naoise_thing (Autodesk Fusion 360 design; units mm, degrees)
Autodesk Fusion 360 part; units mm, degrees
note: some values were not read from the file. Set by a fixed rule: which sketch regions a step uses.
(part 1 of 2)
sketch "Sketch2" plane through (0, 0, 0) normal (0, 0, 1) x (1, 0, 0)
  spline S0 degree 3 poles (35.719, -1.0848) (35.583, -1.8378) (35.7119, -15.8578) (35.8563, -16.002) knots 0 0 0 0 1 1 1 1
  spline S1 degree 3 poles (35.8563, -16.002) (36.0722, -16.2179) (69.5076, -16.2584) (69.8021, -16.0433) knots 0 0 0 0 1 1 1 1
  spline S2 degree 3 poles (69.8021, -16.0433) (70.0037, -15.8956) (70.0088, -15.7107) (70.0088, -8.4275) knots 0 0 0 0 1 1 1 1
  spline S3 degree 3 poles (70.0088, -8.4275) (70.0088, 0.3215) (70.0741, -0.0561) (68.8446, -1.7161) knots 0 0 0 0 1 1 1 1
  spline S4 degree 3 poles (68.8446, -1.7161) (64.4631, -7.6311) (59.6874, -7.6798) (54.1131, -1.8661) knots 0 0 0 0 1 1 1 1
  spline S5 degree 3 poles (54.1131, -1.8661) (53.5197, -1.2472) (52.9609, -0.7408) (52.8712, -0.7408) knots 0 0 0 0 1 1 1 1
  spline S6 degree 3 poles (52.8712, -0.7408) (52.7815, -0.7408) (52.1002, -1.3499) (51.3572, -2.0944) knots 0 0 0 0 1 1 1 1
  spline S7 degree 3 poles (51.3572, -2.0944) (45.7435, -7.7192) (41.5531, -7.6258) (36.9001, -1.7727) knots 0 0 0 0 1 1 1 1
  spline S8 degree 3 poles (36.9001, -1.7727) (36.0177, -0.6628) (35.8166, -0.5456) (35.719, -1.0848) knots 0 0 0 0 1 1 1 1
  spline S9 degree 3 poles (0.635, -11.6292) (0.223, -11.7446) (0.2588, -12.0764) (0.7948, -13.1146) knots 0 0 0 0 1 1 1 1
  spline S10 degree 3 poles (0.7948, -13.1146) (2.1296, -15.6988) (3.7576, -16.9738) (6.2135, -17.3577) knots 0 0 0 0 1 1 1 1
  spline S11 degree 3 poles (6.2135, -17.3577) (7.3075, -17.5289) (7.2747, -17.504) (7.5221, -18.342) knots 0 0 0 0 1 1 1 1
  spline S12 degree 3 poles (7.5221, -18.342) (8.2973, -20.968) (9.7838, -22.1623) (12.7302, -22.5269) knots 0 0 0 0 1 1 1 1
  spline S13 degree 3 poles (12.7302, -22.5269) (13.7266, -22.6502) (13.756, -22.6727) (14.3089, -23.7358) knots 0 0 0 0 1 1 1 1
  spline S14 degree 3 poles (14.3089, -23.7358) (15.7255, -26.4583) (17.1659, -26.9026) (24.6592, -26.9285) knots 0 0 0 0 1 1 1 1
  line L0 (24.6592, -26.9285) -> (29.3687, -26.9449)
  line L1 (29.3688, -26.9449) -> (30.4469, -27.6577)
  spline S15 degree 3 poles (30.4469, -27.6577) (33.8122, -29.8826) (38.332, -30.8367) (42.83, -30.2715) knots 0 0 0 0 1 1 1 1
  spline S16 degree 3 poles (42.83, -30.2715) (44.7186, -30.0342) (44.7204, -29.8995) (42.8464, -29.0565) knots 0 0 0 0 1 1 1 1
  spline S17 degree 3 poles (42.8464, -29.0565) (36.3696, -26.1432) (32.2559, -21.2281) (29.5241, -13.1397) knots 0 0 0 0 1 1 1 1
  spline S18 degree 3 poles (29.5241, -13.1397) (29.2978, -12.4703) (29.0378, -11.8475) (28.9459, -11.7557) knots 0 0 0 0 1 1 1 1
  spline S19 degree 3 poles (28.9459, -11.7557) (28.7689, -11.5784) (1.2562, -11.4557) (0.635, -11.6292) knots 0 0 0 0 1 1 1 1
  spline S20 degree 3 poles (77.0705, -11.611) (76.7252, -11.6771) (76.594, -11.9293) (75.9828, -13.6993) knots 0 0 0 0 1 1 1 1
  spline S21 degree 3 poles (75.9828, -13.6993) (73.2996, -21.4731) (69.0594, -26.361) (62.5277, -29.2105) knots 0 0 0 0 1 1 1 1
  spline S22 degree 3 poles (62.5277, -29.2105) (61.0055, -29.8744) (61.0529, -30.0667) (62.7854, -30.2601) knots 0 0 0 0 1 1 1 1
  spline S23 degree 3 poles (62.7854, -30.2601) (67.6685, -30.8044) (71.9122, -29.9088) (75.3533, -27.6072) knots 0 0 0 0 1 1 1 1
  line L2 (75.3533, -27.6072) -> (76.3588, -26.9346)
  line L3 (76.3588, -26.9346) -> (79.7454, -26.9661)
  spline S24 degree 3 poles (79.7454, -26.9661) (88.0734, -27.0433) (90.0023, -26.4845) (91.503, -23.5596) knots 0 0 0 0 1 1 1 1
  spline S25 degree 3 poles (91.503, -23.5596) (91.9636, -22.6618) (92.044, -22.6121) (93.222, -22.4922) knots 0 0 0 0 1 1 1 1
  spline S26 degree 3 poles (93.222, -22.4922) (95.7363, -22.2366) (97.354, -20.9555) (98.0726, -18.651) knots 0 0 0 0 1 1 1 1
  spline S27 degree 3 poles (98.0726, -18.651) (98.4165, -17.5477) (98.4499, -17.5159) (99.4143, -17.3725) knots 0 0 0 0 1 1 1 1
  spline S28 degree 3 poles (99.4143, -17.3725) (101.9715, -16.9923) (103.7812, -15.5445) (105.0568, -12.8585) knots 0 0 0 0 1 1 1 1
  spline S29 degree 3 poles (105.0568, -12.8585) (105.4714, -11.9854) (105.4783, -11.738) (105.092, -11.6303) knots 0 0 0 0 1 1 1 1
  spline S30 degree 3 poles (105.092, -11.6303) (104.8102, -11.552) (77.4766, -11.5329) (77.0705, -11.611) knots 0 0 0 0 1 1 1 1
  spline S31 degree 3 poles (52.3581, -27.8543) (51.9438, -28.589) (48.2476, -35.5724) (47.3265, -37.3605) knots 0 0 0 0 1 1 1 1
  spline S32 degree 3 poles (47.3265, -37.3605) (46.3479, -39.2607) (46.3468, -39.1938) (47.3644, -39.8854) knots 0 0 0 0 1 1 1 1
  spline S33 degree 3 poles (47.3644, -39.8854) (49.407, -41.2737) (49.8475, -42.7553) (49.8475, -48.2391) knots 0 0 0 0 1 1 1 1
  spline S34 degree 3 poles (49.8475, -48.2391) (49.8475, -52.5754) (49.9795, -52.1877) (48.4182, -52.4357) knots 0 0 0 0 1 1 1 1
  spline S35 degree 3 poles (48.4182, -52.4357) (36.6948, -54.2975) (27.8365, -64.1128) (27.141, -76.0116) knots 0 0 0 0 1 1 1 1
  spline S36 degree 3 poles (27.141, -76.0116) (27.0357, -77.8134) (27.6042, -77.6293) (22.1541, -77.6256) knots 0 0 0 0 1 1 1 1
  spline S37 degree 3 poles (22.1541, -77.6256) (15.6213, -77.6208) (14.2327, -77.2231) (12.8855, -74.9705) knots 0 0 0 0 1 1 1 1
  spline S38 degree 3 poles (12.8855, -74.9705) (12.391, -74.1437) (12.4203, -74.1394) (10.0756, -75.3867) knots 0 0 0 0 1 1 1 1
  spline S39 degree 3 poles (10.0756, -75.3867) (8.9286, -75.9965) (7.3237, -76.8287) (6.5088, -77.2356) knots 0 0 0 0 1 1 1 1
  spline S40 degree 3 poles (6.5088, -77.2356) (4.3691, -78.3042) (0.8178, -80.2058) (0.6506, -80.3727) knots 0 0 0 0 1 1 1 1
  spline S41 degree 3 poles (0.6506, -80.3727) (0.3257, -80.6966) (0.6289, -80.921) (3.3086, -82.3394) knots 0 0 0 0 1 1 1 1
  spline S42 degree 3 poles (3.3086, -82.3394) (4.7776, -83.117) (6.9321, -84.2619) (8.0963, -84.8836) knots 0 0 0 0 1 1 1 1
  spline S43 degree 3 poles (8.0963, -84.8836) (12.5838, -87.2808) (12.3521, -87.2112) (12.8865, -86.3177) knots 0 0 0 0 1 1 1 1
  spline S44 degree 3 poles (12.8865, -86.3177) (13.5485, -85.2106) (14.832, -84.3254) (16.4571, -83.8544) knots 0 0 0 0 1 1 1 1
  spline S45 degree 3 poles (16.4571, -83.8544) (17.5273, -83.544) (27.5381, -83.5073) (27.7995, -83.8126) knots 0 0 0 0 1 1 1 1
  spline S46 degree 3 poles (27.7995, -83.8126) (28.6538, -84.8103) (28.806, -87.4985) (28.1056, -89.2201) knots 0 0 0 0 1 1 1 1
  spline S47 degree 3 poles (28.1056, -89.2201) (27.4325, -90.8748) (27.0375, -93.0585) (27.201, -94.2189) knots 0 0 0 0 1 1 1 1
  spline S48 degree 3 poles (27.201, -94.2189) (27.5804, -96.91) (34.4808, -102.4467) (37.4555, -102.4467) knots 0 0 0 0 1 1 1 1
  spline S49 degree 3 poles (37.4555, -102.4467) (39.3348, -102.4467) (40.9678, -99.7635) (41.8999, -95.1442) knots 0 0 0 0 1 1 1 1
  spline S50 degree 3 poles (41.8999, -95.1442) (42.8593, -90.3891) (42.3669, -88.6473) (39.5851, -86.9574) knots 0 0 0 0 1 1 1 1
  spline S51 degree 3 poles (39.5851, -86.9574) (37.9746, -85.979) (36.8218, -84.2939) (37.3803, -83.7353) knots 0 0 0 0 1 1 1 1
  spline S52 degree 3 poles (37.3803, -83.7353) (37.6208, -83.4948) (49.4525, -83.5589) (49.6723, -83.8017) knots 0 0 0 0 1 1 1 1
  spline S53 degree 3 poles (49.6723, -83.8017) (49.9007, -84.0542) (49.9388, -98.6692) (49.7118, -98.9613) knots 0 0 0 0 1 1 1 1
  spline S54 degree 3 poles (49.7118, -98.9613) (49.6409, -99.0523) (49.1305, -99.4521) (48.5775, -99.8495) knots 0 0 0 0 1 1 1 1
  spline S55 degree 3 poles (48.5775, -99.8495) (42.4288, -104.2681) (38.5662, -110.0365) (37.342, -116.6283) knots 0 0 0 0 1 1 1 1
  spline S56 degree 3 poles (37.342, -116.6283) (37.1642, -117.5861) (37.1652, -121.3281) (37.3436, -122.4492) knots 0 0 0 0 1 1 1 1
  spline S57 degree 3 poles (37.3436, -122.4492) (38.309, -128.5137) (42.2148, -134.9542) (48.2854, -140.4911) knots 0 0 0 0 1 1 1 1
  spline S58 degree 3 poles (48.2854, -140.4911) (49.027, -141.1676) (49.6819, -141.8109) (49.7406, -141.9206) knots 0 0 0 0 1 1 1 1
  spline S59 degree 3 poles (49.7406, -141.9206) (49.938, -142.2892) (49.8811, -158.2782) (49.6792, -159.2564) knots 0 0 0 0 1 1 1 1
  spline S60 degree 3 poles (49.6792, -159.2564) (49.2913, -161.1344) (48.4841, -162.4113) (47.1736, -163.2212) knots 0 0 0 0 1 1 1 1
  spline S61 degree 3 poles (47.1736, -163.2212) (46.291, -163.7665) (46.2367, -163.5546) (48.2158, -167.3032) knots 0 0 0 0 1 1 1 1
  spline S62 degree 3 poles (48.2158, -167.3032) (49.1892, -169.1473) (50.4865, -171.6087) (51.0987, -172.7729) knots 0 0 0 0 1 1 1 1
  spline S63 degree 3 poles (51.0987, -172.7729) (52.682, -175.7839) (52.7915, -175.9355) (53.1043, -175.551) knots 0 0 0 0 1 1 1 1
  spline S64 degree 3 poles (53.1043, -175.551) (53.2855, -175.328) (59.1383, -164.2084) (59.163, -164.0403) knots 0 0 0 0 1 1 1 1
  spline S65 degree 3 poles (59.163, -164.0403) (59.2132, -163.6961) (59.1338, -163.5995) (58.4277, -163.1471) knots 0 0 0 0 1 1 1 1
  spline S66 degree 3 poles (58.4277, -163.1471) (57.6789, -162.6672) (57.0645, -161.9695) (56.6327, -161.109) knots 0 0 0 0 1 1 1 1
  spline S67 degree 3 poles (56.6327, -161.109) (56.2655, -160.3775) (56.3258, -160.1044) (57.0807, -159.0797) knots 0 0 0 0 1 1 1 1
  spline S68 degree 3 poles (57.0807, -159.0797) (58.5393, -157.0993) (59.1905, -155.9229) (59.794, -154.1772) knots 0 0 0 0 1 1 1 1
  spline S69 degree 3 poles (59.794, -154.1772) (61.8601, -148.2013) (60.8065, -143.0586) (56.1922, -136.5957) knots 0 0 0 0 1 1 1 1
  line L4 (56.1922, -136.5957) -> (55.8271, -136.0845)
  line L5 (55.8271, -136.0845) -> (55.8271, -121.144)
  spline S70 degree 3 poles (55.8271, -121.144) (55.8271, -109.8153) (55.8575, -106.1508) (55.9525, -105.9852) knots 0 0 0 0 1 1 1 1
  spline S71 degree 3 poles (55.9525, -105.9852) (56.0774, -105.768) (58.6944, -103.9831) (62.23, -101.7042) knots 0 0 0 0 1 1 1 1
  spline S72 degree 3 poles (62.23, -101.7042) (70.1106, -96.6245) (74.0892, -91.9438) (76.2611, -85.1958) knots 0 0 0 0 1 1 1 1
  spline S73 degree 3 poles (76.2611, -85.1958) (76.835, -83.4139) (76.0812, -83.5922) (82.859, -83.634) knots 0 0 0 0 1 1 1 1
  spline S74 degree 3 poles (82.859, -83.634) (88.5187, -83.6689) (88.6516, -83.6745) (89.4284, -83.911) knots 0 0 0 0 1 1 1 1
  spline S75 degree 3 poles (89.4284, -83.911) (91.0037, -84.3907) (92.093, -85.1551) (92.774, -86.2584) knots 0 0 0 0 1 1 1 1
  spline S76 degree 3 poles (92.774, -86.2584) (93.3916, -87.2591) (92.3584, -87.6665) (101.5214, -82.8074) knots 0 0 0 0 1 1 1 1
  spline S77 degree 3 poles (101.5214, -82.8074) (105.0269, -80.9485) (105.3714, -80.7164) (105.1039, -80.3942) knots 0 0 0 0 1 1 1 1
  spline S78 degree 3 poles (105.1039, -80.3942) (105.0425, -80.3201) (103.6455, -79.5552) (101.9995, -78.694) knots 0 0 0 0 1 1 1 1
  spline S79 degree 3 poles (101.9995, -78.694) (92.4428, -73.6949) (93.3447, -74.0624) (92.8367, -74.9612) knots 0 0 0 0 1 1 1 1
  spline S80 degree 3 poles (92.8367, -74.9612) (91.5382, -77.2589) (89.7731, -77.7116) (82.3156, -77.6594) knots 0 0 0 0 1 1 1 1
  spline S81 degree 3 poles (82.3156, -77.6594) (77.0308, -77.6227) (77.5811, -77.8288) (77.4594, -75.8407) knots 0 0 0 0 1 1 1 1
  spline S82 degree 3 poles (77.4594, -75.8407) (76.7593, -64.4001) (68.4755, -54.9127) (57.1704, -52.6031) knots 0 0 0 0 1 1 1 1
  spline S83 degree 3 poles (57.1704, -52.6031) (55.7048, -52.3039) (55.8266, -52.6957) (55.8308, -48.2822) knots 0 0 0 0 1 1 1 1
  spline S84 degree 3 poles (55.8308, -48.2822) (55.8358, -42.7199) (56.4335, -40.885) (58.6317, -39.6811) knots 0 0 0 0 1 1 1 1
  spline S85 degree 3 poles (58.6317, -39.6811) (59.4778, -39.2176) (59.8609, -40.1143) (54.4724, -29.9508) knots 0 0 0 0 1 1 1 1
  spline S86 degree 3 poles (54.4724, -29.9508) (52.9656, -27.1084) (52.8458, -26.9896) (52.3581, -27.8543) knots 0 0 0 0 1 1 1 1
  spline S87 degree 3 poles (49.6811, -63.1373) (49.9203, -63.3762) (49.9356, -77.0972) (49.6972, -77.4234) knots 0 0 0 0 1 1 1 1
  spline S88 degree 3 poles (49.6972, -77.4234) (49.5041, -77.6877) (37.2189, -77.8021) (36.7242, -77.5441) knots 0 0 0 0 1 1 1 1
  spline S89 degree 3 poles (36.7242, -77.5441) (35.9989, -77.166) (36.9401, -73.3586) (38.3775, -70.8554) knots 0 0 0 0 1 1 1 1
  spline S90 degree 3 poles (57.8908, -63.6773) (63.0642, -65.5854) (67.0576, -70.3741) (68.0736, -75.8881) knots 0 0 0 0 1 1 1 1
  spline S91 degree 3 poles (68.0736, -75.8881) (68.321, -77.2313) (68.2993, -77.421) (67.881, -77.5801) knots 0 0 0 0 1 1 1 1
  spline S92 degree 3 poles (67.881, -77.5801) (67.3201, -77.7933) (56.2385, -77.6624) (56.016, -77.4398) knots 0 0 0 0 1 1 1 1
  spline S93 degree 3 poles (56.016, -77.4398) (55.7551, -77.179) (55.7197, -63.6619) (55.979, -63.3495) knots 0 0 0 0 1 1 1 1
  spline S94 degree 3 poles (55.979, -63.3495) (56.1729, -63.1158) (56.5393, -63.1788) (57.8908, -63.6773) knots 0 0 0 0 1 1 1 1
  spline S95 degree 3 poles (67.3095, -83.7663) (67.6767, -84.2089) (65.918, -87.6308) (64.3448, -89.535) knots 0 0 0 0 1 1 1 1
  spline S96 degree 3 poles (57.4818, -94.9415) (56.1676, -95.6654) (56.0155, -95.6757) (55.8543, -95.0534) knots 0 0 0 0 1 1 1 1
  spline S97 degree 3 poles (55.8543, -95.0534) (55.6953, -94.4396) (55.8046, -83.9851) (55.9723, -83.7832) knots 0 0 0 0 1 1 1 1
  spline S98 degree 3 poles (55.9723, -83.7832) (56.1827, -83.5298) (67.0997, -83.5136) (67.3095, -83.7663) knots 0 0 0 0 1 1 1 1
  spline S99 degree 3 poles (47.0956, -117.9573) (47.6329, -115.5229) (49.1337, -112.3511) (49.6647, -112.5281) knots 0 0 0 0 1 1 1 1
  spline S100 degree 3 poles (49.6647, -112.5281) (49.7655, -112.5617) (49.8007, -114.3624) (49.8218, -120.5659) knots 0 0 0 0 1 1 1 1
  line L6 (0, -88.0004) -> (0, -176.0008)
  line L7 (0, -176.0008) -> (52.9167, -176.0008)
  line L8 (52.9167, -176.0008) -> (105.8333, -176.0008)
  line L9 (105.8333, -176.0008) -> (105.8333, -88.0004)
  line L10 (105.8333, -88.0004) -> (105.8333, 0)
  line L11 (105.8333, 0) -> (52.9167, 0)
  line L12 (52.9167, 0) -> (0, 0)
  line L13 (0, 0) -> (0, -88.0004)
  spline S101 degree 3 poles (36.9001, -1.7727) (41.5531, -7.6258) (45.7435, -7.7192) (51.3572, -2.0944) knots 0 0 0 0 1 1 1 1
  spline S102 degree 3 poles (51.3572, -2.0944) (52.1002, -1.3499) (52.7815, -0.7408) (52.8712, -0.7408) knots 0 0 0 0 1 1 1 1
  spline S103 degree 3 poles (52.8712, -0.7408) (52.9609, -0.7408) (53.5197, -1.2472) (54.1131, -1.8661) knots 0 0 0 0 1 1 1 1
  spline S104 degree 3 poles (54.1131, -1.8661) (59.6874, -7.6798) (64.4631, -7.6311) (68.8446, -1.7161) knots 0 0 0 0 1 1 1 1
  spline S105 degree 3 poles (68.8446, -1.7161) (70.0741, -0.0561) (70.0088, 0.3215) (70.0088, -8.4275) knots 0 0 0 0 1 1 1 1
  spline S106 degree 3 poles (70.0088, -8.4275) (70.0088, -15.7107) (70.0037, -15.8956) (69.8021, -16.0433) knots 0 0 0 0 1 1 1 1
  spline S107 degree 3 poles (69.8021, -16.0433) (69.5076, -16.2584) (36.0722, -16.2179) (35.8563, -16.002) knots 0 0 0 0 1 1 1 1
  spline S108 degree 3 poles (35.8563, -16.002) (35.7119, -15.8578) (35.583, -1.8378) (35.719, -1.0848) knots 0 0 0 0 1 1 1 1
  spline S109 degree 3 poles (35.719, -1.0848) (35.8166, -0.5456) (36.0177, -0.6628) (36.9001, -1.7727) knots 0 0 0 0 1 1 1 1
  spline S110 degree 3 poles (28.9459, -11.7557) (29.0378, -11.8475) (29.2978, -12.4703) (29.5241, -13.1397) knots 0 0 0 0 1 1 1 1
  spline S111 degree 3 poles (29.5241, -13.1397) (32.2559, -21.2281) (36.3696, -26.1432) (42.8464, -29.0565) knots 0 0 0 0 1 1 1 1
  spline S112 degree 3 poles (42.8464, -29.0565) (44.7204, -29.8995) (44.7186, -30.0342) (42.83, -30.2715) knots 0 0 0 0 1 1 1 1
  spline S113 degree 3 poles (42.83, -30.2715) (38.332, -30.8367) (33.8122, -29.8826) (30.4469, -27.6577) knots 0 0 0 0 1 1 1 1
  line L14 (30.4469, -27.6577) -> (29.3688, -26.9449)
  line L15 (29.3688, -26.9449) -> (24.6592, -26.9285)
  spline S114 degree 3 poles (24.6592, -26.9285) (17.1659, -26.9026) (15.7255, -26.4583) (14.3089, -23.7358) knots 0 0 0 0 1 1 1 1
  spline S115 degree 3 poles (14.3089, -23.7358) (13.756, -22.6727) (13.7266, -22.6502) (12.7302, -22.5269) knots 0 0 0 0 1 1 1 1
  spline S116 degree 3 poles (12.7302, -22.5269) (9.7838, -22.1623) (8.2973, -20.968) (7.5221, -18.342) knots 0 0 0 0 1 1 1 1
  spline S117 degree 3 poles (7.5221, -18.342) (7.2747, -17.504) (7.3075, -17.5289) (6.2135, -17.3577) knots 0 0 0 0 1 1 1 1
  spline S118 degree 3 poles (6.2135, -17.3577) (3.7576, -16.9738) (2.1296, -15.6988) (0.7948, -13.1146) knots 0 0 0 0 1 1 1 1
  spline S119 degree 3 poles (0.7948, -13.1146) (0.2588, -12.0764) (0.223, -11.7446) (0.635, -11.6292) knots 0 0 0 0 1 1 1 1
  spline S120 degree 3 poles (0.635, -11.6292) (1.2562, -11.4557) (28.7689, -11.5784) (28.9459, -11.7557) knots 0 0 0 0 1 1 1 1
  spline S121 degree 3 poles (105.092, -11.6303) (105.4783, -11.738) (105.4714, -11.9854) (105.0568, -12.8585) knots 0 0 0 0 1 1 1 1
  spline S122 degree 3 poles (105.0568, -12.8585) (103.7812, -15.5445) (101.9715, -16.9923) (99.4143, -17.3725) knots 0 0 0 0 1 1 1 1
  spline S123 degree 3 poles (99.4143, -17.3725) (98.4499, -17.5159) (98.4165, -17.5477) (98.0726, -18.651) knots 0 0 0 0 1 1 1 1
  spline S124 degree 3 poles (98.0726, -18.651) (97.354, -20.9555) (95.7363, -22.2366) (93.222, -22.4922) knots 0 0 0 0 1 1 1 1
  spline S125 degree 3 poles (93.222, -22.4922) (92.044, -22.6121) (91.9636, -22.6618) (91.503, -23.5596) knots 0 0 0 0 1 1 1 1
  spline S126 degree 3 poles (91.503, -23.5596) (90.0023, -26.4845) (88.0734, -27.0433) (79.7454, -26.9661) knots 0 0 0 0 1 1 1 1
  line L16 (79.7454, -26.9661) -> (76.3588, -26.9346)
  line L17 (76.3588, -26.9346) -> (75.3533, -27.6072)
  spline S127 degree 3 poles (75.3533, -27.6072) (71.9122, -29.9088) (67.6685, -30.8044) (62.7854, -30.2601) knots 0 0 0 0 1 1 1 1
  spline S128 degree 3 poles (62.7854, -30.2601) (61.0529, -30.0667) (61.0055, -29.8744) (62.5277, -29.2105) knots 0 0 0 0 1 1 1 1
  spline S129 degree 3 poles (62.5277, -29.2105) (69.0594, -26.361) (73.2996, -21.4731) (75.9828, -13.6993) knots 0 0 0 0 1 1 1 1
  spline S130 degree 3 poles (75.9828, -13.6993) (76.594, -11.9293) (76.7252, -11.6771) (77.0705, -11.611) knots 0 0 0 0 1 1 1 1
  spline S131 degree 3 poles (77.0705, -11.611) (77.4766, -11.5329) (104.8102, -11.552) (105.092, -11.6303) knots 0 0 0 0 1 1 1 1
  spline S132 degree 3 poles (54.4724, -29.9508) (59.8609, -40.1143) (59.4778, -39.2176) (58.6317, -39.6811) knots 0 0 0 0 1 1 1 1
  spline S133 degree 3 poles (58.6317, -39.6811) (56.4335, -40.885) (55.8358, -42.7199) (55.8308, -48.2822) knots 0 0 0 0 1 1 1 1
  spline S134 degree 3 poles (55.8308, -48.2822) (55.8266, -52.6957) (55.7048, -52.3039) (57.1704, -52.6031) knots 0 0 0 0 1 1 1 1
  spline S135 degree 3 poles (57.1704, -52.6031) (68.4755, -54.9127) (76.7593, -64.4001) (77.4594, -75.8407) knots 0 0 0 0 1 1 1 1
  spline S136 degree 3 poles (77.4594, -75.8407) (77.5811, -77.8288) (77.0308, -77.6227) (82.3156, -77.6594) knots 0 0 0 0 1 1 1 1
  spline S137 degree 3 poles (82.3156, -77.6594) (89.7731, -77.7116) (91.5382, -77.2589) (92.8367, -74.9612) knots 0 0 0 0 1 1 1 1
  spline S138 degree 3 poles (92.8367, -74.9612) (93.3447, -74.0624) (92.4428, -73.6949) (101.9995, -78.694) knots 0 0 0 0 1 1 1 1
  spline S139 degree 3 poles (101.9995, -78.694) (103.6455, -79.5552) (105.0425, -80.3201) (105.1039, -80.3942) knots 0 0 0 0 1 1 1 1
  spline S140 degree 3 poles (105.1039, -80.3942) (105.3714, -80.7164) (105.0269, -80.9485) (101.5214, -82.8074) knots 0 0 0 0 1 1 1 1
  spline S141 degree 3 poles (101.5214, -82.8074) (92.3584, -87.6665) (93.3916, -87.2591) (92.774, -86.2584) knots 0 0 0 0 1 1 1 1
  spline S142 degree 3 poles (92.774, -86.2584) (92.093, -85.1551) (91.0037, -84.3907) (89.4284, -83.911) knots 0 0 0 0 1 1 1 1
  spline S143 degree 3 poles (89.4284, -83.911) (88.6516, -83.6745) (88.5187, -83.6689) (82.859, -83.634) knots 0 0 0 0 1 1 1 1
  spline S144 degree 3 poles (82.859, -83.634) (76.0812, -83.5922) (76.835, -83.4139) (76.2611, -85.1958) knots 0 0 0 0 1 1 1 1
  spline S145 degree 3 poles (76.2611, -85.1958) (74.0892, -91.9438) (70.1106, -96.6245) (62.23, -101.7042) knots 0 0 0 0 1 1 1 1
  spline S146 degree 3 poles (62.23, -101.7042) (58.6944, -103.9831) (56.0774, -105.768) (55.9525, -105.9852) knots 0 0 0 0 1 1 1 1
  spline S147 degree 3 poles (55.9525, -105.9852) (55.8575, -106.1508) (55.8271, -109.8153) (55.8271, -121.144) knots 0 0 0 0 1 1 1 1
  line L18 (55.8271, -121.144) -> (55.8271, -136.0845)
  line L19 (55.8271, -136.0845) -> (56.1922, -136.5957)
  spline S148 degree 3 poles (56.1922, -136.5957) (60.8065, -143.0586) (61.8601, -148.2013) (59.794, -154.1772) knots 0 0 0 0 1 1 1 1
  spline S149 degree 3 poles (59.794, -154.1772) (59.1905, -155.9229) (58.5393, -157.0993) (57.0807, -159.0797) knots 0 0 0 0 1 1 1 1
  spline S150 degree 3 poles (57.0807, -159.0797) (56.3258, -160.1044) (56.2655, -160.3775) (56.6327, -161.109) knots 0 0 0 0 1 1 1 1
  spline S151 degree 3 poles (56.6327, -161.109) (57.0645, -161.9695) (57.6789, -162.6672) (58.4277, -163.1471) knots 0 0 0 0 1 1 1 1
  spline S152 degree 3 poles (58.4277, -163.1471) (59.1338, -163.5995) (59.2132, -163.6961) (59.163, -164.0403) knots 0 0 0 0 1 1 1 1
  spline S153 degree 3 poles (59.163, -164.0403) (59.1383, -164.2084) (53.2855, -175.328) (53.1043, -175.551) knots 0 0 0 0 1 1 1 1
  spline S154 degree 3 poles (53.1043, -175.551) (52.7915, -175.9355) (52.682, -175.7839) (51.0987, -172.7729) knots 0 0 0 0 1 1 1 1
  spline S155 degree 3 poles (51.0987, -172.7729) (50.4865, -171.6087) (49.1892, -169.1473) (48.2158, -167.3032) knots 0 0 0 0 1 1 1 1
  spline S156 degree 3 poles (48.2158, -167.3032) (46.2367, -163.5546) (46.291, -163.7665) (47.1736, -163.2212) knots 0 0 0 0 1 1 1 1
  spline S157 degree 3 poles (47.1736, -163.2212) (48.4841, -162.4113) (49.2913, -161.1344) (49.6792, -159.2564) knots 0 0 0 0 1 1 1 1
  spline S158 degree 3 poles (49.6792, -159.2564) (49.8811, -158.2782) (49.938, -142.2892) (49.7406, -141.9206) knots 0 0 0 0 1 1 1 1
  spline S159 degree 3 poles (49.7406, -141.9206) (49.6819, -141.8109) (49.027, -141.1676) (48.2854, -140.4911) knots 0 0 0 0 1 1 1 1
  spline S160 degree 3 poles (48.2854, -140.4911) (42.2148, -134.9542) (38.309, -128.5137) (37.3436, -122.4492) knots 0 0 0 0 1 1 1 1
  spline S161 degree 3 poles (37.3436, -122.4492) (37.1652, -121.3281) (37.1642, -117.5861) (37.342, -116.6283) knots 0 0 0 0 1 1 1 1
  spline S162 degree 3 poles (37.342, -116.6283) (38.5662, -110.0365) (42.4288, -104.2681) (48.5775, -99.8495) knots 0 0 0 0 1 1 1 1
  spline S163 degree 3 poles (48.5775, -99.8495) (49.1305, -99.4521) (49.6409, -99.0523) (49.7118, -98.9613) knots 0 0 0 0 1 1 1 1
  spline S164 degree 3 poles (49.7118, -98.9613) (49.9388, -98.6692) (49.9007, -84.0542) (49.6723, -83.8017) knots 0 0 0 0 1 1 1 1
  spline S165 degree 3 poles (49.6723, -83.8017) (49.4525, -83.5589) (37.6208, -83.4948) (37.3803, -83.7353) knots 0 0 0 0 1 1 1 1
  spline S166 degree 3 poles (37.3803, -83.7353) (36.8218, -84.2939) (37.9746, -85.979) (39.5851, -86.9574) knots 0 0 0 0 1 1 1 1
  spline S167 degree 3 poles (39.5851, -86.9574) (42.3669, -88.6473) (42.8593, -90.3891) (41.8999, -95.1442) knots 0 0 0 0 1 1 1 1
  spline S168 degree 3 poles (41.8999, -95.1442) (40.9678, -99.7635) (39.3348, -102.4467) (37.4555, -102.4467) knots 0 0 0 0 1 1 1 1
  spline S169 degree 3 poles (37.4555, -102.4467) (34.4808, -102.4467) (27.5804, -96.91) (27.201, -94.2189) knots 0 0 0 0 1 1 1 1
  spline S170 degree 3 poles (27.201, -94.2189) (27.0375, -93.0585) (27.4325, -90.8748) (28.1056, -89.2201) knots 0 0 0 0 1 1 1 1
  spline S171 degree 3 poles (28.1056, -89.2201) (28.806, -87.4985) (28.6538, -84.8103) (27.7995, -83.8126) knots 0 0 0 0 1 1 1 1
  spline S172 degree 3 poles (27.7995, -83.8126) (27.5381, -83.5073) (17.5273, -83.544) (16.4571, -83.8544) knots 0 0 0 0 1 1 1 1
  spline S173 degree 3 poles (16.4571, -83.8544) (14.832, -84.3254) (13.5485, -85.2106) (12.8865, -86.3177) knots 0 0 0 0 1 1 1 1
  spline S174 degree 3 poles (12.8865, -86.3177) (12.3521, -87.2112) (12.5838, -87.2808) (8.0963, -84.8836) knots 0 0 0 0 1 1 1 1
  spline S175 degree 3 poles (8.0963, -84.8836) (6.9321, -84.2619) (4.7776, -83.117) (3.3086, -82.3394) knots 0 0 0 0 1 1 1 1
  spline S176 degree 3 poles (3.3086, -82.3394) (0.6289, -80.921) (0.3257, -80.6966) (0.6506, -80.3727) knots 0 0 0 0 1 1 1 1
  spline S177 degree 3 poles (0.6506, -80.3727) (0.8178, -80.2058) (4.3691, -78.3042) (6.5088, -77.2356) knots 0 0 0 0 1 1 1 1
  spline S178 degree 3 poles (6.5088, -77.2356) (7.3237, -76.8287) (8.9286, -75.9965) (10.0756, -75.3867) knots 0 0 0 0 1 1 1 1
  spline S179 degree 3 poles (10.0756, -75.3867) (12.4203, -74.1394) (12.391, -74.1437) (12.8855, -74.9705) knots 0 0 0 0 1 1 1 1
  spline S180 degree 3 poles (12.8855, -74.9705) (14.2327, -77.2231) (15.6213, -77.6208) (22.1541, -77.6256) knots 0 0 0 0 1 1 1 1
  spline S181 degree 3 poles (22.1541, -77.6256) (27.6042, -77.6293) (27.0357, -77.8134) (27.141, -76.0116) knots 0 0 0 0 1 1 1 1
  spline S182 degree 3 poles (27.141, -76.0116) (27.8365, -64.1128) (36.6948, -54.2975) (48.4182, -52.4357) knots 0 0 0 0 1 1 1 1
  spline S183 degree 3 poles (48.4182, -52.4357) (49.9795, -52.1877) (49.8475, -52.5754) (49.8475, -48.2391) knots 0 0 0 0 1 1 1 1
  spline S184 degree 3 poles (49.8475, -48.2391) (49.8475, -42.7553) (49.407, -41.2737) (47.3644, -39.8854) knots 0 0 0 0 1 1 1 1
  spline S185 degree 3 poles (47.3644, -39.8854) (46.3468, -39.1938) (46.3479, -39.2607) (47.3265, -37.3605) knots 0 0 0 0 1 1 1 1
  spline S186 degree 3 poles (47.3265, -37.3605) (48.2476, -35.5724) (51.9438, -28.589) (52.3581, -27.8543) knots 0 0 0 0 1 1 1 1
  spline S187 degree 3 poles (52.3581, -27.8543) (52.8458, -26.9896) (52.9656, -27.1084) (54.4724, -29.9508) knots 0 0 0 0 1 1 1 1
  spline S188 degree 3 poles (48.8421, -63.0425) (44.6177, -63.9855) (40.5995, -66.9856) (38.3775, -70.8554) knots 0 0 0 0 1 1 1 1
  spline S189 degree 3 poles (38.3775, -70.8554) (36.9401, -73.3586) (35.9989, -77.166) (36.7242, -77.5441) knots 0 0 0 0 1 1 1 1
  spline S190 degree 3 poles (36.7242, -77.5441) (37.2189, -77.8021) (49.5041, -77.6877) (49.6972, -77.4234) knots 0 0 0 0 1 1 1 1
  spline S191 degree 3 poles (49.6972, -77.4234) (49.9356, -77.0972) (49.9203, -63.3762) (49.6811, -63.1373) knots 0 0 0 0 1 1 1 1
  spline S192 degree 3 poles (55.979, -63.3495) (55.7197, -63.6619) (55.7551, -77.179) (56.016, -77.4398) knots 0 0 0 0 1 1 1 1
  spline S193 degree 3 poles (56.016, -77.4398) (56.2385, -77.6624) (67.3201, -77.7933) (67.881, -77.5801) knots 0 0 0 0 1 1 1 1
  spline S194 degree 3 poles (67.881, -77.5801) (68.2993, -77.421) (68.321, -77.2313) (68.0736, -75.8881) knots 0 0 0 0 1 1 1 1
  spline S195 degree 3 poles (68.0736, -75.8881) (67.0576, -70.3741) (63.0642, -65.5854) (57.8908, -63.6773) knots 0 0 0 0 1 1 1 1
  spline S196 degree 3 poles (57.8908, -63.6773) (56.5393, -63.1788) (56.1729, -63.1158) (55.979, -63.3495) knots 0 0 0 0 1 1 1 1
  spline S197 degree 3 poles (55.9723, -83.7832) (55.8046, -83.9851) (55.6953, -94.4396) (55.8543, -95.0534) knots 0 0 0 0 1 1 1 1
  spline S198 degree 3 poles (55.8543, -95.0534) (56.0155, -95.6757) (56.1676, -95.6654) (57.4818, -94.9415) knots 0 0 0 0 1 1 1 1
  spline S199 degree 3 poles (57.4818, -94.9415) (60.3607, -93.3561) (62.7295, -91.4897) (64.3448, -89.535) knots 0 0 0 0 1 1 1 1
  spline S200 degree 3 poles (64.3448, -89.535) (65.918, -87.6308) (67.6767, -84.2089) (67.3095, -83.7663) knots 0 0 0 0 1 1 1 1
  spline S201 degree 3 poles (67.3095, -83.7663) (67.0997, -83.5136) (56.1827, -83.5298) (55.9723, -83.7832) knots 0 0 0 0 1 1 1 1
  spline S202 degree 3 poles (47.0956, -117.9573) (46.3725, -121.2337) (47.3787, -126.184) (49.2199, -128.4063) knots 0 0 0 0 1 1 1 1
  spline S203 degree 3 poles (49.2199, -128.4063) (49.8703, -129.1913) (49.8517, -129.4323) (49.8218, -120.5659) knots 0 0 0 0 1 1 1 1
  spline S204 degree 5 poles (48.8421, -63.0425) (48.8696, -63.0347) (48.9238, -63.0199) (49.0022, -63.0003) (49.1012, -62.9791) (49.215, -62.9616) (49.3178, -62.9541) (49.4086, -62.9573) (49.4868, -62.9719) (49.5525, -62.9978) (49.6067, -63.0341) (49.6414, -63.0708) (49.663, -63.1025) (49.6754, -63.1254) (49.6811, -63.1373) knots 0 0 0 0 0 0 0.1 0.2 0.3 0.4 0.5 0.6 0.7 0.8 0.9 1 1 1 1 1 1
  point P0 (49.424, -62.9624)
extrude "Extrude3" add sketch "Sketch2" along normal blind 5 contours S0 S1 S2 S3 S4 S5 S6 S7 S8 S101 S102 S103 S104 S105 S106 S107 S108 S109 | S9 S10 S11 S12 S13 S14 L0 L1 S15 S16 S17 S18 S19 S110 S111 S112 S113 L14 L15 S114 S115 S116 S117 S118 S119 S120 | S20 S21 S22 S23 L2 L3 S24 S25 S26 S27 S28 S29 S30 S121 S122 S123 S124 S125 S126 L16 L17 S127 S128 S129 S130 S131 | S31 S32 S33 S34 S35 S36 S37 S38 S39 S40 S41 S42 S43 S44 S45 S46 S47 S48 S49 S50 S51 S52 S53 S54 S55 S56 S57 S58 S59 S60 S61 S62 S63 S64 S65 S66 S67 S68 S69 L4 L5 S70 S71 S72 S73 S74 S75 S76 S77 S78 S79 S80 S81 S82 S83 S84 S85 S86 S132 S133 S134 S135 S136 S137 S138 S139 S140 S141 S142 S143 S144 S145 S146 S147 L18 L19 S148 S149 S150 S151 S152 S153 S154 S155 S156 S157 S158 S159 S160 S161 S162 S163 S164 S165 S166 S167 S168 S169 S170 S171 S172 S173 S174 S175 S176 S177 S178 S179 S180 S181 S182 S183 S184 S185 S186 S187 | S87 S88 S89 S188 S189 S190 S191 S204 | S90 S91 S92 S93 S94 S192 S193 S194 S195 S196 | S95 S96 S97 S98 S197 S198 S199 S200 S201 | S99 S100 S202 S203 | L6 L7 L8 L9 L10 L11 L12 L13
extrude "Extrude4" add sketch "Sketch2" against normal blind 5 contours S0 S1 S2 S3 S4 S5 S6 S7 S8 S101 S102 S103 S104 S105 S106 S107 S108 S109 | S9 S10 S11 S12 S13 S14 L0 L1 S15 S16 S17 S18 S19 S110 S111 S112 S113 L14 L15 S114 S115 S116 S117 S118 S119 S120 | S20 S21 S22 S23 L2 L3 S24 S25 S26 S27 S28 S29 S30 S121 S122 S123 S124 S125 S126 L16 L17 S127 S128 S129 S130 S131 | S31 S32 S33 S34 S35 S36 S37 S38 S39 S40 S41 S42 S43 S44 S45 S46 S47 S48 S49 S50 S51 S52 S53 S54 S55 S56 S57 S58 S59 S60 S61 S62 S63 S64 S65 S66 S67 S68 S69 L4 L5 S70 S71 S72 S73 S74 S75 S76 S77 S78 S79 S80 S81 S82 S83 S84 S85 S86 S132 S133 S134 S135 S136 S137 S138 S139 S140 S141 S142 S143 S144 S145 S146 S147 L18 L19 S148 S149 S150 S151 S152 S153 S154 S155 S156 S157 S158 S159 S160 S161 S162 S163 S164 S165 S166 S167 S168 S169 S170 S171 S172 S173 S174 S175 S176 S177 S178 S179 S180 S181 S182 S183 S184 S185 S186 S187
sketch "Sketch1" plane through (0, 0, 0) normal (0, 0, 1) x (1, 0, 0)
  spline S0 degree 3 poles (69.269, -1.1364) (64.5999, -7.5856) (60.1218, -7.8928) (54.4221, -2.155) knots 0 0 0 0 1 1 1 1
  spline S1 degree 3 poles (54.4221, -2.155) (53.6493, -1.3772) (52.9484, -0.7408) (52.8648, -0.7408) knots 0 0 0 0 1 1 1 1
  spline S2 degree 3 poles (52.8648, -0.7408) (52.7809, -0.7408) (52.0552, -1.3957) (51.2519, -2.196) knots 0 0 0 0 1 1 1 1
  spline S3 degree 3 poles (51.2519, -2.196) (45.4721, -7.9547) (41.0363, -7.5716) (36.2418, -0.8996) knots 0 0 0 0 1 1 1 1
  spline S4 degree 3 poles (36.2418, -0.8996) (36.0915, -0.6903) (35.9688, -0.6178) (35.845, -0.6654) knots 0 0 0 0 1 1 1 1
  spline S5 degree 3 poles (35.845, -0.6654) (35.556, -0.7763) (35.5703, -15.7557) (35.8598, -16.0176) knots 0 0 0 0 1 1 1 1
  spline S6 degree 3 poles (35.8598, -16.0176) (36.0389, -16.1798) (37.3428, -16.1912) (52.9783, -16.1663) knots 0 0 0 0 1 1 1 1
  line L0 (52.9783, -16.1663) -> (69.9029, -16.1396)
  line L1 (69.9029, -16.1396) -> (69.9302, -8.432)
  spline S7 degree 3 poles (69.9302, -8.432) (69.945, -4.1929) (69.9191, -0.6562) (69.8722, -0.5726) knots 0 0 0 0 1 1 1 1
  spline S8 degree 3 poles (69.8722, -0.5726) (69.809, -0.4593) (69.6542, -0.6038) (69.269, -1.1364) knots 0 0 0 0 1 1 1 1
  spline S9 degree 3 poles (0.3895, -11.6049) (-0.0087, -12.0031) (1.4354, -14.5944) (2.6895, -15.7319) knots 0 0 0 0 1 1 1 1
  spline S10 degree 3 poles (2.6895, -15.7319) (3.7658, -16.7079) (4.7678, -17.1106) (7.1562, -17.5263) knots 0 0 0 0 1 1 1 1
  spline S11 degree 3 poles (7.1562, -17.5263) (7.3361, -17.5578) (7.4038, -17.6861) (7.5012, -18.1808) knots 0 0 0 0 1 1 1 1
  spline S12 degree 3 poles (7.5012, -18.1808) (7.9909, -20.6693) (9.9171, -22.2901) (12.6357, -22.5007) knots 0 0 0 0 1 1 1 1
  spline S13 degree 3 poles (12.6357, -22.5007) (13.5938, -22.575) (13.9115, -22.7182) (14.0129, -23.1219) knots 0 0 0 0 1 1 1 1
  spline S14 degree 3 poles (14.0129, -23.1219) (14.1581, -23.7014) (14.9812, -24.9028) (15.5575, -25.3767) knots 0 0 0 0 1 1 1 1
  spline S15 degree 3 poles (15.5575, -25.3767) (17.1723, -26.7052) (18.4248, -26.9126) (24.7306, -26.8975) knots 0 0 0 0 1 1 1 1
  line L2 (24.7306, -26.8975) -> (29.2997, -26.8864)
  line L3 (29.2997, -26.8864) -> (29.8106, -27.2497)
  spline S16 degree 3 poles (29.8106, -27.2497) (32.9634, -29.4918) (35.7145, -30.316) (40.0579, -30.3194) knots 0 0 0 0 1 1 1 1
  spline S17 degree 3 poles (40.0579, -30.3194) (44.414, -30.3228) (45.2914, -30.0892) (43.5838, -29.3801) knots 0 0 0 0 1 1 1 1
  spline S18 degree 3 poles (43.5838, -29.3801) (37.9415, -27.0378) (34.2127, -23.4484) (31.3137, -17.5683) knots 0 0 0 0 1 1 1 1
  spline S19 degree 3 poles (31.3137, -17.5683) (30.6739, -16.2706) (29.442, -13.1133) (29.2698, -12.3296) knots 0 0 0 0 1 1 1 1
  spline S20 degree 3 poles (29.2698, -12.3296) (29.0899, -11.5112) (30.6292, -11.5922) (14.6725, -11.5607) knots 0 0 0 0 1 1 1 1
  spline S21 degree 3 poles (14.6725, -11.5607) (6.8564, -11.5454) (0.4292, -11.5652) (0.3895, -11.6049) knots 0 0 0 0 1 1 1 1
  spline S22 degree 3 poles (76.8728, -11.6409) (76.7001, -11.7105) (76.5514, -12.0187) (76.2508, -12.9305) knots 0 0 0 0 1 1 1 1
  spline S23 degree 3 poles (76.2508, -12.9305) (73.3494, -21.73) (69.2838, -26.3223) (61.4124, -29.6913) knots 0 0 0 0 1 1 1 1
  spline S24 degree 3 poles (61.4124, -29.6913) (60.5256, -30.071) (62.0784, -30.3096) (65.4579, -30.313) knots 0 0 0 0 1 1 1 1
  spline S25 degree 3 poles (65.4579, -30.313) (69.9151, -30.3178) (72.2596, -29.6741) (75.4002, -27.5833) knots 0 0 0 0 1 1 1 1
  line L4 (75.4002, -27.5833) -> (76.4524, -26.883)
  line L5 (76.4524, -26.883) -> (81.1207, -26.8909)
  spline S26 degree 3 poles (81.1207, -26.8909) (88.5933, -26.9034) (90.083, -26.4216) (91.512, -23.5302) knots 0 0 0 0 1 1 1 1
  spline S27 degree 3 poles (91.512, -23.5302) (91.9718, -22.5999) (91.9853, -22.5909) (93.0865, -22.5031) knots 0 0 0 0 1 1 1 1
  spline S28 degree 3 poles (93.0865, -22.5031) (95.7905, -22.2874) (97.4016, -20.9629) (98.1583, -18.3332) knots 0 0 0 0 1 1 1 1
  spline S29 degree 3 poles (98.1583, -18.3332) (98.3888, -17.5329) (98.4015, -17.5149) (98.7533, -17.4853) knots 0 0 0 0 1 1 1 1
  spline S30 degree 3 poles (98.7533, -17.4853) (100.8745, -17.3069) (102.7287, -16.3229) (103.909, -14.7495) knots 0 0 0 0 1 1 1 1
  spline S31 degree 3 poles (103.909, -14.7495) (104.6898, -13.7091) (105.5777, -11.8967) (105.4076, -11.6917) knots 0 0 0 0 1 1 1 1
  spline S32 degree 3 poles (105.4076, -11.6917) (105.2597, -11.5133) (77.3118, -11.4636) (76.8728, -11.6409) knots 0 0 0 0 1 1 1 1
  spline S33 degree 3 poles (52.7431, -27.282) (52.6251, -27.3561) (50.5595, -31.1893) (47.8139, -36.4289) knots 0 0 0 0 1 1 1 1
  spline S34 degree 3 poles (47.8139, -36.4289) (46.2941, -39.3293) (46.301, -39.3009) (47.0408, -39.6814) knots 0 0 0 0 1 1 1 1
  spline S35 degree 3 poles (47.0408, -39.6814) (48.1534, -40.2537) (49.1487, -41.6332) (49.6025, -43.2329) knots 0 0 0 0 1 1 1 1
  spline S36 degree 3 poles (49.6025, -43.2329) (49.8528, -44.1156) (49.9496, -51.9594) (49.7126, -52.156) knots 0 0 0 0 1 1 1 1
  spline S37 degree 3 poles (49.7126, -52.156) (49.6311, -52.2237) (49.1987, -52.3298) (48.7519, -52.392) knots 0 0 0 0 1 1 1 1
  spline S38 degree 3 poles (48.7519, -52.392) (36.9477, -54.0337) (27.791, -64.0667) (27.1399, -76.0722) knots 0 0 0 0 1 1 1 1
  spline S39 degree 3 poles (27.1399, -76.0722) (27.0433, -77.8558) (27.5323, -77.6822) (22.6142, -77.6785) knots 0 0 0 0 1 1 1 1
  spline S40 degree 3 poles (22.6142, -77.6785) (15.8591, -77.6732) (14.1848, -77.2218) (12.9593, -75.0761) knots 0 0 0 0 1 1 1 1
  spline S41 degree 3 poles (12.9593, -75.0761) (12.4047, -74.1053) (12.4833, -74.1238) (11.389, -74.7054) knots 0 0 0 0 1 1 1 1
  spline S42 degree 3 poles (11.389, -74.7054) (8.8527, -76.0529) (7.0197, -77.0035) (6.7723, -77.0996) knots 0 0 0 0 1 1 1 1
  spline S43 degree 3 poles (6.7723, -77.0996) (6.6225, -77.1578) (5.2874, -77.8478) (3.8055, -78.6328) knots 0 0 0 0 1 1 1 1
  spline S44 degree 3 poles (3.8055, -78.6328) (2.3236, -79.4179) (0.9684, -80.1322) (0.7938, -80.2203) knots 0 0 0 0 1 1 1 1
  spline S45 degree 3 poles (0.7938, -80.2203) (0.0415, -80.5998) (0.317, -80.8035) (4.5291, -82.9839) knots 0 0 0 0 1 1 1 1
  spline S46 degree 3 poles (4.5291, -82.9839) (5.5597, -83.5173) (6.5458, -84.0372) (6.7204, -84.1391) knots 0 0 0 0 1 1 1 1
  spline S47 degree 3 poles (6.7204, -84.1391) (7.094, -84.3571) (10.0155, -85.9115) (11.367, -86.6114) knots 0 0 0 0 1 1 1 1
  spline S48 degree 3 poles (11.367, -86.6114) (12.4336, -87.1635) (12.4172, -87.1667) (12.8929, -86.3248) knots 0 0 0 0 1 1 1 1
  spline S49 degree 3 poles (12.8929, -86.3248) (13.3088, -85.589) (14.1057, -84.8667) (14.9963, -84.4182) knots 0 0 0 0 1 1 1 1
  spline S50 degree 3 poles (14.9963, -84.4182) (16.4767, -83.6729) (16.4042, -83.6806) (22.3155, -83.6359) knots 0 0 0 0 1 1 1 1
  spline S51 degree 3 poles (22.3155, -83.6359) (28.1699, -83.5919) (27.9556, -83.57) (28.0763, -84.2232) knots 0 0 0 0 1 1 1 1
  spline S52 degree 3 poles (28.0763, -84.2232) (28.1054, -84.3799) (28.2525, -84.9842) (28.4035, -85.5662) knots 0 0 0 0 1 1 1 1
  spline S53 degree 3 poles (28.4035, -85.5662) (28.8041, -87.109) (28.7433, -87.72) (28.0133, -89.4821) knots 0 0 0 0 1 1 1 1
  spline S54 degree 3 poles (28.0133, -89.4821) (27.1865, -91.4784) (26.9311, -94.0615) (27.4521, -95.1627) knots 0 0 0 0 1 1 1 1
  spline S55 degree 3 poles (27.4521, -95.1627) (28.8152, -98.0443) (35.3695, -102.6597) (37.7494, -102.4141) knots 0 0 0 0 1 1 1 1
  spline S56 degree 3 poles (37.7494, -102.4141) (39.5137, -102.2321) (41.053, -99.4722) (41.9521, -94.8796) knots 0 0 0 0 1 1 1 1
  spline S57 degree 3 poles (41.9521, -94.8796) (42.8604, -90.2401) (42.3894, -88.6656) (39.583, -86.959) knots 0 0 0 0 1 1 1 1
  spline S58 degree 3 poles (39.583, -86.959) (38.1947, -86.115) (36.93, -84.4338) (37.1843, -83.7708) knots 0 0 0 0 1 1 1 1
  spline S59 degree 3 poles (37.1843, -83.7708) (37.2671, -83.5552) (49.5059, -83.5208) (49.7205, -83.7353) knots 0 0 0 0 1 1 1 1
  spline S60 degree 3 poles (49.7205, -83.7353) (49.8557, -83.8705) (49.9155, -98.5478) (49.7821, -98.8952) knots 0 0 0 0 1 1 1 1
  spline S61 degree 3 poles (49.7821, -98.8952) (49.7464, -98.9888) (49.3059, -99.3476) (48.8032, -99.6926) knots 0 0 0 0 1 1 1 1
  spline S62 degree 3 poles (48.8032, -99.6926) (45.3491, -102.0646) (41.8846, -105.8058) (39.9915, -109.2092) knots 0 0 0 0 1 1 1 1
  spline S63 degree 3 poles (39.9915, -109.2092) (34.8462, -118.4587) (36.6586, -127.9506) (45.4086, -137.5807) knots 0 0 0 0 1 1 1 1
  spline S64 degree 3 poles (45.4086, -137.5807) (46.6587, -138.9565) (46.708, -139.0068) (47.8991, -140.1167) knots 0 0 0 0 1 1 1 1
  spline S65 degree 3 poles (47.8991, -140.1167) (48.3013, -140.4914) (48.9058, -141.0576) (49.2424, -141.3753) knots 0 0 0 0 1 1 1 1
  line L6 (49.2424, -141.3753) -> (49.8546, -141.9529)
  line L7 (49.8546, -141.9529) -> (49.8221, -150.5365)
  spline S66 degree 3 poles (49.8221, -150.5365) (49.7861, -160.0983) (49.824, -159.5882) (49.0379, -161.1585) knots 0 0 0 0 1 1 1 1
  spline S67 degree 3 poles (49.0379, -161.1585) (48.5891, -162.0554) (47.8713, -162.827) (47.0469, -163.2984) knots 0 0 0 0 1 1 1 1
  spline S68 degree 3 poles (47.0469, -163.2984) (46.3145, -163.7176) (46.314, -163.7715) (47.0273, -165.0725) knots 0 0 0 0 1 1 1 1
  spline S69 degree 3 poles (47.0273, -165.0725) (47.3387, -165.6406) (47.9171, -166.7245) (48.3127, -167.4813) knots 0 0 0 0 1 1 1 1
  spline S70 degree 3 poles (48.3127, -167.4813) (48.7079, -168.238) (49.1604, -169.0952) (49.3178, -169.3863) knots 0 0 0 0 1 1 1 1
  spline S71 degree 3 poles (49.3178, -169.3863) (49.5795, -169.8699) (49.9213, -170.5192) (51.463, -173.4608) knots 0 0 0 0 1 1 1 1
  spline S72 degree 3 poles (51.463, -173.4608) (53.0103, -176.4133) (52.6619, -176.4948) (54.6367, -172.72) knots 0 0 0 0 1 1 1 1
  spline S73 degree 3 poles (54.6367, -172.72) (55.2585, -171.5315) (57.7532, -166.806) (58.6962, -165.0315) knots 0 0 0 0 1 1 1 1
  spline S74 degree 3 poles (58.6962, -165.0315) (59.4098, -163.6879) (59.4135, -163.7297) (58.5343, -163.2074) knots 0 0 0 0 1 1 1 1
  spline S75 degree 3 poles (58.5343, -163.2074) (57.6546, -162.6846) (57.1582, -162.1306) (56.6502, -161.1037) knots 0 0 0 0 1 1 1 1
  spline S76 degree 3 poles (56.6502, -161.1037) (56.1975, -160.1888) (56.1684, -160.2917) (57.3225, -158.7447) knots 0 0 0 0 1 1 1 1
  spline S77 degree 3 poles (57.3225, -158.7447) (62.1768, -152.2381) (61.9141, -144.4395) (56.5968, -137.2021) knots 0 0 0 0 1 1 1 1
  line L8 (56.5968, -137.2021) -> (55.8271, -136.1546)
  line L9 (55.8271, -136.1546) -> (55.8271, -121.1159)
  spline S78 degree 3 poles (55.8271, -121.1159) (55.8271, -108.7729) (55.8522, -106.0471) (55.9676, -105.9082) knots 0 0 0 0 1 1 1 1
  spline S79 degree 3 poles (55.9676, -105.9082) (56.0448, -105.8151) (57.1402, -105.0539) (58.4017, -104.2167) knots 0 0 0 0 1 1 1 1
  spline S80 degree 3 poles (58.4017, -104.2167) (67.3627, -98.2694) (67.3505, -98.2782) (69.433, -96.2041) knots 0 0 0 0 1 1 1 1
  spline S81 degree 3 poles (69.433, -96.2041) (72.5048, -93.1447) (74.9771, -89.1794) (76.1971, -85.3546) knots 0 0 0 0 1 1 1 1
  spline S82 degree 3 poles (76.1971, -85.3546) (76.6884, -83.8144) (76.7334, -83.7171) (76.9818, -83.6546) knots 0 0 0 0 1 1 1 1
  spline S83 degree 3 poles (76.9818, -83.6546) (77.1062, -83.6237) (79.8028, -83.6144) (82.9747, -83.6343) knots 0 0 0 0 1 1 1 1
  line L10 (82.9747, -83.6343) -> (88.7412, -83.6702)
  line L11 (88.7412, -83.6702) -> (89.5879, -83.9528)
  spline S84 degree 3 poles (89.5879, -83.9528) (91.1524, -84.4748) (92.189, -85.2466) (92.8299, -86.3661) knots 0 0 0 0 1 1 1 1
  spline S85 degree 3 poles (92.8299, -86.3661) (93.3381, -87.2543) (92.9315, -87.4064) (99.4833, -83.8771) knots 0 0 0 0 1 1 1 1
  spline S86 degree 3 poles (99.4833, -83.8771) (100.2691, -83.4538) (101.5788, -82.7611) (102.3938, -82.3381) knots 0 0 0 0 1 1 1 1
  spline S87 degree 3 poles (102.3938, -82.3381) (105.745, -80.5974) (105.7077, -80.6349) (104.6393, -80.0828) knots 0 0 0 0 1 1 1 1
  spline S88 degree 3 poles (104.6393, -80.0828) (104.3355, -79.9259) (103.6585, -79.5695) (103.1346, -79.2906) knots 0 0 0 0 1 1 1 1
  spline S89 degree 3 poles (103.1346, -79.2906) (99.9744, -77.6097) (99.3873, -77.3033) (98.3721, -76.8059) knots 0 0 0 0 1 1 1 1
  spline S90 degree 3 poles (98.3721, -76.8059) (97.9646, -76.6061) (96.7139, -75.9595) (95.5926, -75.3689) knots 0 0 0 0 1 1 1 1
  spline S91 degree 3 poles (95.5926, -75.3689) (93.2386, -74.1288) (93.2545, -74.1323) (92.9434, -74.7731) knots 0 0 0 0 1 1 1 1
  spline S92 degree 3 poles (92.9434, -74.7731) (91.7713, -77.185) (89.9986, -77.6809) (82.5437, -77.6814) knots 0 0 0 0 1 1 1 1
  spline S93 degree 3 poles (82.5437, -77.6814) (76.9906, -77.6817) (77.5457, -77.8626) (77.4586, -76.0235) knots 0 0 0 0 1 1 1 1
  spline S94 degree 3 poles (77.4586, -76.0235) (77.1673, -69.8738) (74.462, -63.8392) (70.017, -59.4236) knots 0 0 0 0 1 1 1 1
  spline S95 degree 3 poles (70.017, -59.4236) (66.6218, -56.0509) (62.0858, -53.6252) (57.3394, -52.6436) knots 0 0 0 0 1 1 1 1
  spline S96 degree 3 poles (57.3394, -52.6436) (56.624, -52.4957) (55.9911, -52.3274) (55.9329, -52.2698) knots 0 0 0 0 1 1 1 1
  spline S97 degree 3 poles (55.9329, -52.2698) (55.6953, -52.0335) (55.8157, -44.5034) (56.0737, -43.4578) knots 0 0 0 0 1 1 1 1
  spline S98 degree 3 poles (56.0737, -43.4578) (56.5007, -41.7282) (57.4249, -40.3505) (58.5674, -39.7404) knots 0 0 0 0 1 1 1 1
  spline S99 degree 3 poles (58.5674, -39.7404) (59.3881, -39.3023) (59.3881, -39.2528) (58.5711, -37.7021) knots 0 0 0 0 1 1 1 1
  spline S100 degree 3 poles (58.5711, -37.7021) (58.1803, -36.9604) (57.6225, -35.9013) (57.3315, -35.3483) knots 0 0 0 0 1 1 1 1
  spline S101 degree 3 poles (57.3315, -35.3483) (56.5094, -33.786) (55.9797, -32.794) (55.7213, -32.3321) knots 0 0 0 0 1 1 1 1
  spline S102 degree 3 poles (55.7213, -32.3321) (55.5908, -32.0992) (55.1378, -31.242) (54.7142, -30.4271) knots 0 0 0 0 1 1 1 1
  spline S103 degree 3 poles (54.7142, -30.4271) (53.123, -27.3645) (52.9786, -27.1338) (52.7431, -27.282) knots 0 0 0 0 1 1 1 1
  spline S104 degree 3 poles (49.68, -63.0351) (49.9422, -63.1357) (49.9345, -77.1983) (49.6723, -77.4883) knots 0 0 0 0 1 1 1 1
  spline S105 degree 3 poles (49.6723, -77.4883) (49.5065, -77.6716) (49.1622, -77.6817) (43.0707, -77.6817) knots 0 0 0 0 1 1 1 1
  spline S106 degree 3 poles (43.0707, -77.6817) (35.6994, -77.6817) (36.3355, -77.7809) (36.4495, -76.6479) knots 0 0 0 0 1 1 1 1
  spline S107 degree 3 poles (36.4495, -76.6479) (36.8538, -72.6318) (39.2954, -68.4837) (42.7919, -65.8717) knots 0 0 0 0 1 1 1 1
  spline S108 degree 3 poles (42.7919, -65.8717) (44.9088, -64.2903) (48.7881, -62.6928) (49.68, -63.0351) knots 0 0 0 0 1 1 1 1
  spline S109 degree 3 poles (57.3945, -63.5074) (63.0415, -65.3928) (67.3222, -70.5326) (68.1733, -76.4492) knots 0 0 0 0 1 1 1 1
  spline S110 degree 3 poles (68.1733, -76.4492) (68.3006, -77.3345) (68.2969, -77.3949) (68.1064, -77.534) knots 0 0 0 0 1 1 1 1
  spline S111 degree 3 poles (68.1064, -77.534) (67.8035, -77.7555) (56.3356, -77.7531) (56.0324, -77.5314) knots 0 0 0 0 1 1 1 1
  spline S112 degree 3 poles (56.0324, -77.5314) (55.7906, -77.3546) (55.6453, -63.8323) (55.8808, -63.3928) knots 0 0 0 0 1 1 1 1
  spline S113 degree 3 poles (55.8808, -63.3928) (56.0324, -63.1095) (56.2533, -63.1264) (57.3945, -63.5074) knots 0 0 0 0 1 1 1 1
  spline S114 degree 3 poles (67.3846, -83.7853) (67.5283, -84.16) (66.4985, -86.4103) (65.4315, -88.0533) knots 0 0 0 0 1 1 1 1
  spline S115 degree 3 poles (65.4315, -88.0533) (63.8069, -90.5547) (61.0941, -92.9397) (57.7929, -94.769) knots 0 0 0 0 1 1 1 1
  spline S116 degree 3 poles (57.7929, -94.769) (56.0615, -95.7281) (56.029, -95.7379) (55.8885, -95.3341) knots 0 0 0 0 1 1 1 1
  spline S117 degree 3 poles (55.8885, -95.3341) (55.7398, -94.9079) (55.7295, -84.2687) (55.8774, -83.8798) knots 0 0 0 0 1 1 1 1
  line L12 (55.8774, -83.8798) -> (55.9805, -83.6083)
  line L13 (55.9805, -83.6083) -> (61.6487, -83.6083)
  spline S118 degree 3 poles (61.6487, -83.6083) (66.8496, -83.6083) (67.3222, -83.6229) (67.3846, -83.7853) knots 0 0 0 0 1 1 1 1
  spline S119 degree 3 poles (49.8475, -120.65) (49.8475, -129.8977) (49.8811, -129.5381) (49.1273, -128.3465) knots 0 0 0 0 1 1 1 1
  spline S120 degree 3 poles (49.1273, -128.3465) (46.4241, -124.0732) (46.1055, -118.8273) (48.2843, -114.4588) knots 0 0 0 0 1 1 1 1
  spline S121 degree 3 poles (48.2843, -114.4588) (49.9353, -111.148) (49.8475, -110.7998) (49.8475, -120.65) knots 0 0 0 0 1 1 1 1
  line L14 (0, -88.0004) -> (0, -176.0008)
  line L15 (0, -176.0008) -> (52.9167, -176.0008)
  line L16 (52.9167, -176.0008) -> (105.8333, -176.0008)
  line L17 (105.8333, -176.0008) -> (105.8333, -88.0004)
  line L18 (105.8333, -88.0004) -> (105.8333, 0)
  line L19 (105.8333, 0) -> (52.9167, 0)
  line L20 (52.9167, 0) -> (0, 0)
  line L21 (0, 0) -> (0, -88.0004)
  line L22 (69.9302, -8.432) -> (69.9029, -16.1396)
  line L23 (69.9029, -16.1396) -> (52.9783, -16.1663)
  spline S122 degree 3 poles (52.9783, -16.1663) (37.3428, -16.1912) (36.0389, -16.1798) (35.8598, -16.0176) knots 0 0 0 0 1 1 1 1
  spline S123 degree 3 poles (35.8598, -16.0176) (35.5703, -15.7557) (35.556, -0.7763) (35.845, -0.6654) knots 0 0 0 0 1 1 1 1
  spline S124 degree 3 poles (35.845, -0.6654) (35.9688, -0.6178) (36.0915, -0.6903) (36.2418, -0.8996) knots 0 0 0 0 1 1 1 1
  spline S125 degree 3 poles (36.2418, -0.8996) (41.0363, -7.5716) (45.4721, -7.9547) (51.2519, -2.196) knots 0 0 0 0 1 1 1 1
  spline S126 degree 3 poles (51.2519, -2.196) (52.0552, -1.3957) (52.7809, -0.7408) (52.8648, -0.7408) knots 0 0 0 0 1 1 1 1
  spline S127 degree 3 poles (52.8648, -0.7408) (52.9484, -0.7408) (53.6493, -1.3772) (54.4221, -2.155) knots 0 0 0 0 1 1 1 1
  spline S128 degree 3 poles (54.4221, -2.155) (60.1218, -7.8928) (64.5999, -7.5856) (69.269, -1.1364) knots 0 0 0 0 1 1 1 1
  spline S129 degree 3 poles (69.269, -1.1364) (69.6542, -0.6038) (69.809, -0.4593) (69.8722, -0.5726) knots 0 0 0 0 1 1 1 1
  spline S130 degree 3 poles (69.8722, -0.5726) (69.9191, -0.6562) (69.945, -4.1929) (69.9302, -8.432) knots 0 0 0 0 1 1 1 1
  spline S131 degree 3 poles (29.0417, -11.8004) (29.1288, -11.9168) (29.2314, -12.155) (29.2698, -12.3296) knots 0 0 0 0 1 1 1 1
  spline S132 degree 3 poles (29.2698, -12.3296) (29.442, -13.1133) (30.6739, -16.2706) (31.3137, -17.5683) knots 0 0 0 0 1 1 1 1
  spline S133 degree 3 poles (31.3137, -17.5683) (34.2127, -23.4484) (37.9415, -27.0378) (43.5838, -29.3801) knots 0 0 0 0 1 1 1 1
  spline S134 degree 3 poles (43.5838, -29.3801) (45.2914, -30.0892) (44.414, -30.3228) (40.0579, -30.3194) knots 0 0 0 0 1 1 1 1
  spline S135 degree 3 poles (40.0579, -30.3194) (35.7145, -30.316) (32.9634, -29.4918) (29.8106, -27.2497) knots 0 0 0 0 1 1 1 1
  line L24 (29.8106, -27.2497) -> (29.2997, -26.8864)
  line L25 (29.2997, -26.8864) -> (24.7306, -26.8975)
  spline S136 degree 3 poles (24.7306, -26.8975) (18.4248, -26.9126) (17.1723, -26.7052) (15.5575, -25.3767) knots 0 0 0 0 1 1 1 1
  spline S137 degree 3 poles (15.5575, -25.3767) (14.9812, -24.9028) (14.1581, -23.7014) (14.0129, -23.1219) knots 0 0 0 0 1 1 1 1
  spline S138 degree 3 poles (14.0129, -23.1219) (13.9115, -22.7182) (13.5938, -22.575) (12.6357, -22.5007) knots 0 0 0 0 1 1 1 1
  spline S139 degree 3 poles (12.6357, -22.5007) (9.9171, -22.2901) (7.9909, -20.6693) (7.5012, -18.1808) knots 0 0 0 0 1 1 1 1